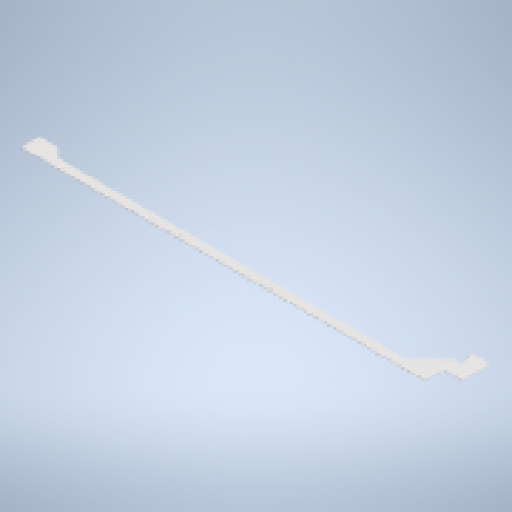
# Autodesk Inventor part: BSH 022 rib floor 2
Saved by Autodesk Inventor 2025 (Build 290162010, 162A)
## iProperties
Created: 2024-07-23
Part Number: BSH 022 rib floor 2
Material: 09g2s
Document SubType Name: Sheet Metal
Designer: admin
Stock Number: БШК 021 шпангоут пол
Mass: 3788.77 g
Surface Area: 3392.95 cm^2
Volume: 482.646 cm^3
Density: 7.85 g/cm^3
Flat Pattern Width: 230 cm
Flat Pattern Length: 25.5463 cm
Flat Pattern Area: 5875.65 cm^2
Sheet Metal Rule: AISI304 3mm Die 32
Sheet Metal Width: 2300,000 mm
Sheet Metal Length: 255,463 mm
Sheet Metal Area: 587564,906 mm^2
Appearance: Default
Author: admin
Autodesk Inventor part; units mm, degrees
ref_plane "YZ Plane" through (0, 0, 0) normal (1, 0, 0) x (0, 1, 0)
ref_plane "XZ Plane" through (0, 0, 0) normal (0, 1, 0) x (-1, 0, 0)
ref_plane "XY Plane" through (0, 0, 0) normal (0, 0, 1) x (1, 0, 0)
sketch "Sketch1" plane through (0, 0, 0) normal (0, 0, 1) x (1, 0, 0)
  line L0 (1200, 2900) -> (-1200, 2900)
  line L1 (-1200, 2900) -> (-1200, 0)
  line L2 (-1200, 0) -> (1200, 0)
  line L3 (1200, 0) -> (1200, 2900)
  line L4 (1150, 2900) -> (1150, 0)
  line L5 (-1150, 0) -> (-1150, 2900) construction
  line L6 (0, 2900) -> (0, 50) construction
  line L7 (-1100, 200.463) -> (-949.537, 50)
  line L8 (-1200, 100) -> (-1100, 100)
  line L9 (-1100, 100) -> (-1100, 0)
  line L10 (-1100, 200.463) -> (-1150, 2900)
  arc A0 (-1100.463, 225.4587) -> (-1082.3223, 182.7853) centre (-1100, 200.463) ccw
  arc A1 (-1082.3223, 182.7853) -> (-1100.463, 225.4587) centre (-1100, 200.463) ccw construction
  line L11 (-1200, 255.463) -> (-1101.0187, 255.463)
  line L12 (0, 50) -> (-949.537, 50)
  line L13 (0, 50) -> (0, 0)
  line L14 (1504.8819, -225.894) -> (355.3449, -225.894)
  dimension "d3" = 2400
  dimension "d4" = 2900
  dimension "d5" = 50
  dimension "d6" = 100
  dimension "d7" = 50
  dimension "d8" = 2644.537
  dimension "d9" = 135
  dimension "d10" = 949.537
  dimension "d11" = 1149.537
  dimension "d12" = 136.061
  dimension "d13" = 50
  dimension "d14" = 100
  dimension "d15" = 212.7868
  dimension "d16" = 2700
  dimension "d17" = 55
  measures "d3" distance of L3.start L1.end
  measures "d4" distance of L1.end L1.start
  measures "d5" diameter of A0
  measures "d6" distance of L8.start L8.end
  measures "d7" distance between parallel lines of L1 L5
  measures "d8" distance between parallel lines of L0 L11
  measures "d9" angle of L12 L7
  measures "d10" distance of L6.end L7.end
  measures "d11" distance of L14.start L14.end
  measures "d12" angle of L7 L10
  measures "d13" distance between parallel lines of L2 L12
  measures "d14" distance from line of L1 L10.start
  measures "d15" distance of L10.start L7.end
  measures "d16" distance of L10.start L10.end
  measures "d17" vertical distance of L10.start L11.end
extrude "Plate1" add sketch "Sketch1" against normal blind 3 contours L10 A0 L7 L12 L13 L2 L9 L8 L1 L11
sketch "Sketch2" plane through (0, 0, 0) normal (0, 0, 1) x (1, 0, 0)
  line L0 (-1100, 0) -> (0, 0) projected
  line L1 (-750.1, 0) -> (-746.9, 0)
  line L2 (-746.9, 0) -> (-746.9, 26)
  line L3 (-746.9, 26) -> (-750.1, 26)
  line L4 (-750.1, 26) -> (-750.1, 0)
  point P0 (-748.5, 0)
  point P1 (-746.9, 0)
  dimension "d20" = 3.2
  dimension "d21" = 26
  dimension "d22" = 748.5
  constraints: 8 end point, 2 parallel, 1 horizontal, 1 horizontal alignment, 1 midpoint, 1 perpendicular, 1 point on line
  measures "d20" distance of L2.end L3.end
  measures "d21" distance of L3.end L1.start
  measures "d22" distance of L0.end point (-748.5, 0)
extrude "Extrusion1" cut sketch "Sketch2" against normal through all
mirror "Mirror2" about plane through (0, 0, 0) normal (1, 0, 0) of "Plate1"
pattern_linear "Rectangular Pattern3" count 5 spacing 500 along (1, 0, 0) of "Extrusion1"
sketch "Sketch3" plane through (0, 0, -3) normal (0, 0, -1) x (-1, 0, 0)
  line L0 (1081.7131, 17.4301) -> (945.1402, 17.4301) construction
  line L1 (945.1402, 17.4301) -> (945.1402, 29.8362) construction
  line L2 (945.1402, 29.8362) -> (1081.7131, 29.8362) construction
  line L3 (1081.7131, 29.8362) -> (1081.7131, 17.4301) construction
  point P0 (0, 0)
  constraints: 2 other
mark "Mark1"
sketch "Sketch4" plane through (949.537, 50, -3) normal (0, 0, -1) x (-1, 0, 0)
  line L0 (2049.537, 50) -> (2049.537, -50) projected
  line L1 (2149.537, 50) -> (2049.537, 50) projected
  line L2 (1899.074, 0) -> (2031.8593, 132.7853) projected
  arc A0 (2031.8593, 132.7853) -> (2050, 175.4587) centre (2049.537, 150.463) ccw projected
  line L3 (2050, 175.4587) -> (2050.5557, 205.463) projected
  line L4 (2050.5557, 205.463) -> (2149.537, 205.463) projected
  line L5 (2149.537, 205.463) -> (2149.537, 50) projected
  line L6 (2049.537, 50) -> (1949.074, 50)
  point P0 (949.537, -50)
  constraints: 2 end point, 1 horizontal, 1 point on line
extrude "Extrusion2" cut sketch "Sketch4" against normal blind 10
equation "\"d11\" = d10 + d18"
equation "\"d14\" = d6"
equation "\"d2\" = Thickness"
equation "\"BendReliefWidth\" = Thickness"
equation "\"BendReliefDepth\" = 0.5 * Thickness"
equation "\"CornerReliefSize\" = 4 * Thickness"
equation "\"MinimumRemnant\" = 2 * Thickness"
equation "\"TransitionRadius\" = BendRadius"
equation "\"JacobiRadiusSize\" = BendRadius"
equation "\"GapSize\" = Thickness"
equation "\"d18\" = d19"
equation "\"Thickness\" = 3"
equation "\"BendRadius\" = 5"
equation "\"d19\" = 200"
body "Solid1"
